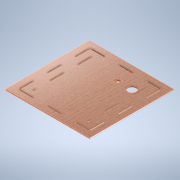
# Autodesk Inventor part: Roof_V2
Saved by Autodesk Inventor 2022.2 (Build 262287000, 287)
## iProperties
Created: 2022-11-15
Part Number: Roof_V2
Material: Generic
Document SubType Name: Modeling
Designer: jaege
Density: 1 g/cm^3
Appearance: Red Oak - Natural Low Gloss
Mass: 344.053 g
Surface Area: 1843.39 cm^2
Volume: 344.053 cm^3
Author: jaege
Autodesk Inventor part; units mm, degrees
(part 1 of 2)
ref_plane "YZ Plane" through (0, 0, 0) normal (1, 0, 0) x (0, 1, 0)
ref_plane "XZ Plane" through (0, 0, 0) normal (0, 1, 0) x (-1, 0, 0)
ref_plane "XY Plane" through (0, 0, 0) normal (0, 0, 1) x (1, 0, 0)
sketch "Sketch1" plane through (0, 0, 0) normal (0, 0, 1) x (1, 0, 0)
  line L0 (120, -66) -> (20, -66) construction
  line L1 (20, -66) -> (20, -26) construction
  line L2 (20, -26) -> (120, -26) construction
  line L3 (120, -26) -> (120, -66) construction
  line L4 (-275, -71) -> (125, -71) construction
  line L5 (125, -71) -> (125, 329) construction
  line L6 (125, 329) -> (-275, 329) construction
  line L7 (-275, 329) -> (-275, -71) construction
  line L8 (50, 104) -> (50, 154) construction
  line L9 (50, 154) -> (54, 154) construction
  line L10 (54, 154) -> (54, 104) construction
  line L11 (54, 104) -> (50, 104) construction
  line L12 (-50, 254) -> (-100, 254) construction
  line L13 (-100, 254) -> (-100, 258) construction
  line L14 (-100, 258) -> (-50, 258) construction
  line L15 (-50, 258) -> (-50, 254) construction
  line L16 (50, 258) -> (50, 254) construction
  line L17 (50, 254) -> (54, 254) construction
  line L18 (54, 254) -> (54, 204) construction
  line L19 (54, 204) -> (50, 204) construction
  line L20 (50, 204) -> (50, 254) construction
  line L21 (50, 254) -> (0, 254) construction
  line L22 (0, 254) -> (0, 258) construction
  line L23 (0, 258) -> (50, 258) construction
  line L24 (54, 4) -> (50, 4) construction
  line L25 (50, 4) -> (50, 0) construction
  line L26 (50, 0) -> (0, 0) construction
  line L27 (0, 0) -> (0, 4) construction
  line L28 (0, 4) -> (50, 4) construction
  line L29 (50, 4) -> (50, 54) construction
  line L30 (50, 54) -> (54, 54) construction
  line L31 (54, 54) -> (54, 4) construction
  line L32 (-100, 4) -> (-50, 4) construction
  line L33 (-50, 4) -> (-50, 0) construction
  line L34 (-50, 0) -> (-100, 0) construction
  line L35 (-100, 0) -> (-100, 4) construction
  line L36 (-204, 254) -> (-200, 254) construction
  line L37 (-200, 254) -> (-200, 258) construction
  line L38 (-200, 258) -> (-150, 258) construction
  line L39 (-150, 258) -> (-150, 254) construction
  line L40 (-150, 254) -> (-200, 254) construction
  line L41 (-200, 254) -> (-200, 204) construction
  line L42 (-200, 204) -> (-204, 204) construction
  line L43 (-204, 204) -> (-204, 254) construction
  line L44 (-200, 154) -> (-200, 104) construction
  line L45 (-200, 104) -> (-204, 104) construction
  line L46 (-204, 104) -> (-204, 154) construction
  line L47 (-204, 154) -> (-200, 154) construction
  line L48 (-200, 54) -> (-200, 4) construction
  line L49 (-200, 4) -> (-150, 4) construction
  line L50 (-150, 4) -> (-150, 0) construction
  line L51 (-150, 0) -> (-200, 0) construction
  line L52 (-200, 0) -> (-200, 4) construction
  line L53 (-200, 4) -> (-204, 4) construction
  line L54 (-204, 4) -> (-204, 54) construction
  line L55 (-204, 54) -> (-200, 54) construction
  line L56 (-275, -71) -> (125, -71) construction
  line L57 (125, -71) -> (125, 329) construction
  line L58 (125, 329) -> (-275, 329) construction
  line L59 (-275, 329) -> (-275, -71) construction
  line L60 (-275, -71) -> (125, 329) construction
  line L61 (75, 279) -> (-225, 279)
  line L62 (-225, 279) -> (-225, -21)
  line L63 (-225, -21) -> (75, -21)
  line L64 (75, -21) -> (75, 279)
  line L65 (75, 279) -> (-225, -21) construction
  line L66 (-225, 279) -> (75, -21) construction
  line L67 (-204, 4) -> (-200, 4)
  line L68 (-200, 4) -> (-200, 54)
  line L69 (-200, 54) -> (-204, 54)
  line L70 (-204, 54) -> (-204, 4)
  line L71 (-200, 104) -> (-204, 104)
  line L72 (-204, 104) -> (-204, 154)
  line L73 (-204, 154) -> (-200, 154)
  line L74 (-200, 154) -> (-200, 104)
  line L75 (-200, 204) -> (-204, 204)
  line L76 (-204, 204) -> (-204, 254)
  line L77 (-204, 254) -> (-200, 254)
  line L78 (-200, 254) -> (-200, 204)
  line L79 (-200, 254) -> (-150, 254)
  line L80 (-150, 254) -> (-150, 258)
  line L81 (-150, 258) -> (-200, 258)
  line L82 (-200, 258) -> (-200, 254)
  line L83 (-100, 254) -> (-50, 254)
  line L84 (-50, 254) -> (-50, 258)
  line L85 (-50, 258) -> (-100, 258)
  line L86 (-100, 258) -> (-100, 254)
  line L87 (0, 254) -> (50, 254)
  line L88 (50, 254) -> (50, 258)
  line L89 (50, 258) -> (0, 258)
  line L90 (0, 258) -> (0, 254)
  line L91 (50, 254) -> (54, 254)
  line L92 (54, 254) -> (54, 204)
  line L93 (54, 204) -> (50, 204)
  line L94 (50, 204) -> (50, 254)
  line L95 (54, 154) -> (50, 154)
  line L96 (50, 154) -> (50, 104)
  line L97 (50, 104) -> (54, 104)
  line L98 (54, 104) -> (54, 154)
  line L99 (54, 4) -> (50, 4)
  line L100 (50, 4) -> (50, 54)
  line L101 (50, 54) -> (54, 54)
  line L102 (54, 54) -> (54, 4)
  line L103 (50, 4) -> (0, 4)
  line L104 (0, 4) -> (0, 0)
  line L105 (0, 0) -> (50, 0)
  line L106 (50, 0) -> (50, 4)
  line L107 (-100, 0) -> (-50, 0)
  line L108 (-50, 0) -> (-50, 4)
  line L109 (-50, 4) -> (-100, 4)
  line L110 (-100, 4) -> (-100, 0)
  line L111 (-200, 0) -> (-150, 0)
  line L112 (-150, 0) -> (-150, 4)
  line L113 (-150, 4) -> (-200, 4)
  line L114 (-200, 4) -> (-200, 0)
  point P0 (-75, 129)
  dimension "d0" = 300
  dimension "d1" = 300
  constraints: 118 end point, 28 parallel, 14 horizontal, 14 perpendicular, 3 midpoint
  measures "d0" distance of L63.end L62.end
  measures "d1" distance of L62.end L61.end
extrude "Extrusion1" add sketch "Sketch1" against normal blind 4
sketch "Sketch2" plane through (0, 0, 0) normal (0, 0, 1) x (1, 0, 0)
  line L0 (-175, 234) -> (-171, 234)
  line L1 (-171, 234) -> (-171, 184)
  line L2 (-171, 184) -> (-175, 184)
  line L3 (-175, 184) -> (-175, 234)
  line L4 (-175, 184) -> (-171, 184)
  line L5 (-171, 184) -> (-171, 134)
  line L6 (-171, 134) -> (-175, 134)
  line L7 (-175, 134) -> (-175, 184)
  line L8 (-175, 134) -> (-171, 134)
  line L9 (-171, 134) -> (-171, 84)
  line L10 (-171, 84) -> (-175, 84)
  line L11 (-175, 84) -> (-175, 134)
  line L12 (-200, 254) -> (-200, 204) projected
  line L13 (-150, 254) -> (-200, 254) projected
  line L14 (-175, 84) -> (-171, 84)
  line L15 (-171, 84) -> (-171, 34)
  line L16 (-171, 34) -> (-175, 34)
  line L17 (-175, 34) -> (-175, 84)
  line L18 (-175, 34) -> (-171, 34)
  line L19 (-171, 34) -> (-171, 24)
  line L20 (-171, 24) -> (-175, 24)
  line L21 (-175, 24) -> (-175, 34)
  line L22 (-200, 4) -> (-150, 4) projected
  line L23 (25, 184) -> (21, 184)
  line L24 (21, 184) -> (25, 184)
  line L25 (21, 234) -> (25, 234)
  line L26 (25, 234) -> (25, 184)
  line L27 (21, 184) -> (21, 234)
  line L28 (25, 184) -> (25, 134)
  line L29 (25, 134) -> (21, 134)
  line L30 (21, 134) -> (25, 134)
  line L31 (25, 134) -> (25, 84)
  line L32 (25, 84) -> (21, 84)
  line L33 (21, 84) -> (21, 134)
  line L34 (21, 134) -> (21, 184)
  line L35 (21, 84) -> (25, 84)
  line L36 (25, 84) -> (25, 34)
  line L37 (21, 34) -> (21, 84)
  line L38 (25, 34) -> (21, 34)
  line L39 (21, 34) -> (25, 34)
  line L40 (25, 34) -> (25, 24)
  line L41 (21, 24) -> (21, 34)
  line L42 (25, 24) -> (21, 24)
  circle A0 centre (0, 204) radius 15
  line L43 (50, 254) -> (0, 254) projected
  line L44 (50, 204) -> (50, 254) projected
  point P0 (0, 0)
  point P1 (-173, 234)
  point P2 (-173, 24)
  point P3 (23, 234)
  point P4 (23, 24)
  point P5 (23, 234)
  point P6 (-75, 184)
  dimension "d4" = 4
  dimension "d5" = 50
  dimension "d6" = 4
  dimension "d7" = 50
  dimension "d8" = 4
  dimension "d9" = 50
  dimension "d10" = 25
  dimension "d11" = 20
  dimension "d12" = 4
  dimension "d13" = 50
  dimension "d14" = 4
  dimension "d15" = 20
  dimension "d20" = 196
  dimension "d25" = 30
  dimension "d29" = 50
  dimension "d30" = 50
  constraints: 80 end point, 10 parallel, 6 horizontal, 5 perpendicular, 3 midpoint, 1 centre point, 38 other
  measures "d4" distance of L1.end L2.end
  measures "d5" distance of L0.end L1.end
  measures "d6" distance of L5.end L6.end
  measures "d7" distance of L4.end L5.end
  measures "d8" distance of L9.end L10.end
  measures "d9" distance of L8.end L9.end
  measures "d10" distance from line of L12 L0.start
  measures "d11" distance from line of L13 point (-173, 234)
  measures "d12" distance of L15.end L16.end
  measures "d13" distance of L14.end L15.end
  measures "d14" distance of L19.end L20.end
  measures "d15" distance from line of L22 point (-173, 24)
  measures "d20" distance of L2.end L23.end
  measures "d25" diameter of A0
  measures "d29" distance of L43.end A0.centre
  measures "d30" distance from line of L44 A0.centre
extrude "Extrusion2" cut sketch "Sketch2" against normal blind 10 contours L0 L1 L2 L3 | L6 L9 L10 L11 | L16 L19 L20 L21 | L23 L27 L25 L26 | L31 L32 L33 L29 | L40 L42 L41 L38 | A0
sketch "Sketch3" plane through (0, 0, 0) normal (0, 0, 1) x (1, 0, 0)
  circle A0 centre (-50, 204) radius 6
  line L0 (-50, 254) -> (-100, 254) projected
  circle A1 centre (0, 204) radius 15 projected
  point P0 (0, 0)
  dimension "d31" = 12
  dimension "d32" = 50
  dimension "d33" = 50
  constraints: 1 centre point
  measures "d31" diameter of A0
  measures "d32" distance from line of A0.centre L0
  measures "d33" distance of A1.centre A0.centre
extrude "Extrusion3" cut sketch "Sketch3" against normal through all contours A0
sketch "Sketch4" plane through (0, 0, 0) normal (0, 0, 1) x (1, 0, 0)
  circle A0 centre (-50, 204) radius 6 projected
  line L0 (21, 84) -> (21, 134) projected
  line L1 (21, 134) -> (25, 134) projected
  line L2 (25, 134) -> (25, 84) projected
  line L3 (25, 84) -> (21, 84) projected
  line L4 (-175, 24) -> (-175, 34) projected
  line L5 (-175, 34) -> (-171, 34) projected
  line L6 (-171, 34) -> (-171, 24) projected
  line L7 (-171, 24) -> (-175, 24) projected
  line L8 (21, 24) -> (21, 34) projected
  line L9 (21, 34) -> (25, 34) projected
  line L10 (25, 34) -> (25, 24) projected
  line L11 (25, 24) -> (21, 24) projected
  line L12 (21, 184) -> (21, 234) projected
  line L13 (21, 234) -> (25, 234) projected
  line L14 (25, 234) -> (25, 184) projected
  line L15 (25, 184) -> (21, 184) projected
  line L16 (-175, 84) -> (-175, 134) projected
  line L17 (-175, 134) -> (-171, 134) projected
  line L18 (-171, 134) -> (-171, 84) projected
  line L19 (-171, 84) -> (-175, 84) projected
  line L20 (-175, 184) -> (-175, 234) projected
  line L21 (-175, 234) -> (-171, 234) projected
  line L22 (-171, 234) -> (-171, 184) projected
  line L23 (-171, 184) -> (-175, 184) projected
  circle A1 centre (0, 204) radius 15 projected
  line L24 (-225, 279) -> (-225, -21) projected
  line L25 (-225, -21) -> (75, -21) projected
  line L26 (75, -21) -> (75, 279) projected
  line L27 (75, 279) -> (-225, 279) projected
  line L28 (-100, 0) -> (-100, 4) projected
  line L29 (-100, 4) -> (-50, 4) projected
  line L30 (-50, 4) -> (-50, 0) projected
  line L31 (-50, 0) -> (-100, 0) projected
  line L32 (54, 4) -> (50, 4) projected
  line L33 (50, 4) -> (50, 0) projected
  line L34 (50, 0) -> (0, 0) projected
  line L35 (0, 0) -> (0, 4) projected
  line L36 (0, 4) -> (50, 4) projected
  line L37 (50, 4) -> (50, 54) projected
  line L38 (50, 54) -> (54, 54) projected
  line L39 (54, 54) -> (54, 4) projected
  line L40 (54, 154) -> (54, 104) projected
  line L41 (54, 104) -> (50, 104) projected
  line L42 (50, 104) -> (50, 154) projected
  line L43 (50, 154) -> (54, 154) projected
  line L44 (50, 204) -> (50, 254) projected
  line L45 (50, 254) -> (0, 254) projected
  line L46 (0, 254) -> (0, 258) projected
  line L47 (0, 258) -> (50, 258) projected
  line L48 (50, 258) -> (50, 254) projected
  line L49 (50, 254) -> (54, 254) projected
  line L50 (54, 254) -> (54, 204) projected
  line L51 (54, 204) -> (50, 204) projected
  line L52 (-100, 254) -> (-100, 258) projected
  line L53 (-100, 258) -> (-50, 258) projected
  line L54 (-50, 258) -> (-50, 254) projected
  line L55 (-50, 254) -> (-100, 254) projected
  line L56 (-204, 254) -> (-200, 254) projected
  line L57 (-200, 254) -> (-200, 258) projected
  line L58 (-200, 258) -> (-150, 258) projected
  line L59 (-150, 258) -> (-150, 254) projected
  line L60 (-150, 254) -> (-200, 254) projected
  line L61 (-200, 254) -> (-200, 204) projected
  line L62 (-200, 204) -> (-204, 204) projected
  line L63 (-204, 204) -> (-204, 254) projected
  line L64 (-200, 104) -> (-204, 104) projected
  line L65 (-204, 104) -> (-204, 154) projected
  line L66 (-204, 154) -> (-200, 154) projected
  line L67 (-200, 154) -> (-200, 104) projected
  line L68 (-200, 54) -> (-200, 4) projected
  line L69 (-200, 4) -> (-150, 4) projected
  line L70 (-150, 4) -> (-150, 0) projected
  line L71 (-150, 0) -> (-200, 0) projected
  line L72 (-200, 0) -> (-200, 4) projected
  line L73 (-200, 4) -> (-204, 4) projected
  line L74 (-204, 4) -> (-204, 54) projected
  line L75 (-204, 54) -> (-200, 54) projected
  line L76 (-58.1443, 209.9414) -> (-57.4426, 209.0769)
  line L77 (-57.4426, 209.0769) -> (-57.732, 208.6915)
  line L78 (-57.732, 208.6915) -> (-60.2646, 209.6927)
  spline S0 degree 2 poles (-60.2646, 209.6927) (-60.3488, 209.7261) (-60.425, 209.7304) (-60.4722, 209.7028) knots 0 0 0 1 2 2 2
  spline S1 degree 2 poles (-60.4722, 209.7028) (-60.5537, 209.6515) (-60.6194, 209.7008) knots 0 0 0 1 1 1
  spline S2 degree 2 poles (-60.6194, 209.7008) (-60.6723, 209.7406) (-60.6606, 209.8708) (-60.6002, 209.9513) knots 0 0 0 1 2 2 2
  line L79 (-60.6002, 209.9513) -> (-59.9722, 210.7875)
  spline S3 degree 2 poles (-59.9722, 210.7875) (-59.9134, 210.8659) (-59.8716, 210.8775) knots 0 0 0 1 1 1
  spline S4 degree 2 poles (-59.8716, 210.8775) (-59.8154, 210.895) (-59.7689, 210.86) knots 0 0 0 1 1 1
  spline S5 degree 2 poles (-59.7689, 210.86) (-59.7138, 210.8186) (-59.7218, 210.7286) knots 0 0 0 1 1 1
  spline S6 degree 2 poles (-59.7218, 210.7286) (-59.7319, 210.6534) (-59.7139, 210.5936) (-59.6716, 210.5618) knots 0 0 0 1 2 2 2
  spline S7 degree 2 poles (-59.6716, 210.5618) (-59.6525, 210.5475) (-59.6287, 210.5395) knots 0 0 0 1 1 1
  line L80 (-59.6287, 210.5395) -> (-58.1443, 209.9414)
  line L81 (-59.5923, 211.2936) -> (-59.3157, 211.6619)
  line L82 (-59.3157, 211.6619) -> (-57.367, 210.8708)
  line L83 (-57.367, 210.8708) -> (-56.7066, 210.0571)
  line L84 (-56.7066, 210.0571) -> (-56.9991, 209.6676)
  line L85 (-56.9991, 209.6676) -> (-58.8832, 210.4301)
  line L86 (-58.8832, 210.4301) -> (-59.5923, 211.2936)
  line L87 (-57.6019, 211.1532) -> (-58.0339, 211.3319)
  line L88 (-58.0339, 211.3319) -> (-58.4646, 211.8606)
  spline S8 degree 2 poles (-58.4646, 211.8606) (-58.5154, 211.9252) (-58.5493, 211.9506) knots 0 0 0 1 1 1
  spline S9 degree 2 poles (-58.5493, 211.9506) (-58.6022, 211.9904) (-58.723, 211.9883) (-58.8077, 211.946) knots 0 0 0 1 2 2 2
  spline S10 degree 2 poles (-58.8077, 211.946) (-58.866, 211.9169) (-58.9359, 211.9164) (-58.9697, 211.9419) knots 0 0 0 1 2 2 2
  spline S11 degree 2 poles (-58.9697, 211.9419) (-59.0163, 211.9768) (-59.012, 212.0663) (-58.9643, 212.1298) knots 0 0 0 1 2 2 2
  line L89 (-58.9643, 212.1298) -> (-58.6448, 212.5554)
  spline S12 degree 2 poles (-58.6448, 212.5554) (-58.5892, 212.6295) (-58.5044, 212.6586) (-58.4557, 212.622) knots 0 0 0 1 2 2 2
  spline S13 degree 2 poles (-58.4557, 212.622) (-58.4261, 212.5997) (-58.4124, 212.5431) (-58.4225, 212.4944) knots 0 0 0 1 2 2 2
  spline S14 degree 2 poles (-58.4225, 212.4944) (-58.4469, 212.3869) (-58.4353, 212.3186) knots 0 0 0 1 1 1
  spline S15 degree 2 poles (-58.4353, 212.3186) (-58.4168, 212.1756) (-58.2903, 212.0177) knots 0 0 0 1 1 1
  line L90 (-58.2903, 212.0177) -> (-57.6019, 211.1532)
  line L91 (-56.7345, 213.9981) -> (-55.9742, 214.48)
  line L92 (-55.9742, 214.48) -> (-54.045, 212.5932)
  spline S16 degree 2 poles (-54.045, 212.5932) (-53.9924, 212.545) (-53.9462, 212.5116) knots 0 0 0 1 1 1
  spline S17 degree 2 poles (-53.9462, 212.5116) (-53.9056, 212.4872) (-53.8333, 212.5017) knots 0 0 0 1 1 1
  spline S18 degree 2 poles (-53.8333, 212.5017) (-53.77, 212.5105) (-53.7064, 212.4943) (-53.6838, 212.4585) knots 0 0 0 1 2 2 2
  spline S19 degree 2 poles (-53.6838, 212.4585) (-53.6214, 212.3601) (-53.769, 212.2666) knots 0 0 0 1 1 1
  line L93 (-53.769, 212.2666) -> (-54.7105, 211.6699)
  spline S20 degree 2 poles (-54.7105, 211.6699) (-54.7664, 211.6345) (-54.8711, 211.6465) (-54.8995, 211.6912) knots 0 0 0 1 2 2 2
  spline S21 degree 2 poles (-54.8995, 211.6912) (-54.9236, 211.7292) (-54.9164, 211.7871) (-54.8819, 211.8465) knots 0 0 0 1 2 2 2
  spline S22 degree 2 poles (-54.8819, 211.8465) (-54.8567, 211.8907) (-54.8537, 211.9553) (-54.875, 211.9888) knots 0 0 0 1 2 2 2
  spline S23 degree 2 poles (-54.875, 211.9888) (-54.8962, 212.0224) (-54.9185, 212.0427) knots 0 0 0 1 1 1
  line L94 (-54.9185, 212.0427) -> (-55.1518, 212.2773)
  line L95 (-55.1518, 212.2773) -> (-55.6773, 211.9442)
  line L96 (-55.6773, 211.9442) -> (-55.7676, 212.2004)
  line L97 (-55.7676, 212.2004) -> (-55.345, 212.4683)
  line L98 (-55.345, 212.4683) -> (-56.6661, 213.7813)
  line L99 (-56.6661, 213.7813) -> (-56.7345, 213.9981)
  line L100 (-56.5617, 213.4337) -> (-56.219, 213.1055)
  line L101 (-56.219, 213.1055) -> (-55.7798, 211.6756)
  spline S24 degree 2 poles (-55.7798, 211.6756) (-55.7614, 211.612) (-55.7331, 211.5672) knots 0 0 0 1 1 1
  spline S25 degree 2 poles (-55.7331, 211.5672) (-55.6579, 211.4487) (-55.5135, 211.4681) knots 0 0 0 1 1 1
  line L102 (-55.5135, 211.4681) -> (-55.4288, 211.4779)
  spline S26 degree 2 poles (-55.4288, 211.4779) (-55.3492, 211.4908) (-55.3067, 211.4237) knots 0 0 0 1 1 1
  spline S27 degree 2 poles (-55.3067, 211.4237) (-55.2472, 211.3298) (-55.3836, 211.2433) knots 0 0 0 1 1 1
  line L103 (-55.3836, 211.2433) -> (-55.8621, 210.94)
  spline S28 degree 2 poles (-55.8621, 210.94) (-55.9337, 210.8947) (-56.0511, 210.9018) (-56.0837, 210.9532) knots 0 0 0 1 2 2 2
  spline S29 degree 2 poles (-56.0837, 210.9532) (-56.1177, 211.0069) (-56.0576, 211.0951) knots 0 0 0 1 1 1
  spline S30 degree 2 poles (-56.0576, 211.0951) (-56.002, 211.1805) (-55.9622, 211.2809) (-55.9585, 211.3492) knots 0 0 0 1 2 2 2
  spline S31 degree 2 poles (-55.9585, 211.3492) (-55.9566, 211.46) (-56.0016, 211.6102) knots 0 0 0 1 1 1
  line L104 (-56.0016, 211.6102) -> (-56.5617, 213.4337)
  line L105 (-52.9721, 215.6794) -> (-52.3659, 213.1239)
  spline S32 degree 2 poles (-52.3659, 213.1239) (-52.3457, 213.0389) (-52.3036, 213.0108) knots 0 0 0 1 1 1
  spline S33 degree 2 poles (-52.3036, 213.0108) (-52.2833, 212.9938) (-52.2493, 212.9883) (-52.1594, 212.9878) knots 0 0 0 1 2 2 2
  spline S34 degree 2 poles (-52.1594, 212.9878) (-52.0483, 212.9897) (-52.0257, 212.8944) knots 0 0 0 1 1 1
  spline S35 degree 2 poles (-52.0257, 212.8944) (-52.0123, 212.8377) (-52.0604, 212.7882) knots 0 0 0 1 1 1
  spline S36 degree 2 poles (-52.0604, 212.7882) (-52.0955, 212.7527) (-52.1908, 212.7301) knots 0 0 0 1 1 1
  line L106 (-52.1908, 212.7301) -> (-52.2655, 212.7123)
  line L107 (-52.2655, 212.7123) -> (-53.2367, 212.4819)
  line L108 (-53.2367, 212.4819) -> (-53.2934, 212.4685)
  spline S37 degree 2 poles (-53.2934, 212.4685) (-53.3706, 212.4502) (-53.4697, 212.4892) (-53.4825, 212.5433) knots 0 0 0 1 2 2 2
  spline S38 degree 2 poles (-53.4825, 212.5433) (-53.5033, 212.6309) (-53.4224, 212.68) knots 0 0 0 1 1 1
  spline S39 degree 2 poles (-53.4224, 212.68) (-53.3564, 212.7229) (-53.3357, 212.7387) (-53.3277, 212.7624) knots 0 0 0 1 2 2 2
  spline S40 degree 2 poles (-53.3277, 212.7624) (-53.3099, 212.802) (-53.3282, 212.8793) knots 0 0 0 1 1 1
  line L109 (-53.3282, 212.8793) -> (-53.844, 215.0535)
  spline S41 degree 2 poles (-53.844, 215.0535) (-53.8623, 215.1308) (-53.896, 215.1581) knots 0 0 0 1 1 1
  spline S42 degree 2 poles (-53.896, 215.1581) (-53.9138, 215.1757) (-53.9394, 215.1805) (-54.0171, 215.1866) knots 0 0 0 1 2 2 2
  spline S43 degree 2 poles (-54.0171, 215.1866) (-54.1114, 215.1941) (-54.1328, 215.2843) knots 0 0 0 1 1 1
  spline S44 degree 2 poles (-54.1328, 215.2843) (-54.1456, 215.3384) (-54.0747, 215.4178) (-53.9974, 215.4361) knots 0 0 0 1 2 2 2
  line L110 (-53.9974, 215.4361) -> (-53.9407, 215.4496)
  line L111 (-53.9407, 215.4496) -> (-52.9721, 215.6794)
  spline S45 degree 2 poles (-51.9455, 214.3229) (-51.7405, 214.3416) (-51.5064, 214.3183) (-51.4035, 214.2746) knots 0 0 0 1 2 2 2
  spline S46 degree 2 poles (-51.4035, 214.2746) (-51.2974, 214.2291) (-51.1555, 214.0668) (-51.1305, 213.9612) knots 0 0 0 1 2 2 2
  line L112 (-51.1305, 213.9612) -> (-51.0242, 213.5129)
  spline S47 degree 2 poles (-51.0242, 213.5129) (-51.007, 213.4408) (-50.9607, 213.4518) knots 0 0 0 1 1 1
  spline S48 degree 2 poles (-50.9607, 213.4518) (-50.9452, 213.4555) (-50.9243, 213.4822) (-50.9105, 213.5154) knots 0 0 0 1 2 2 2
  spline S49 degree 2 poles (-50.9105, 213.5154) (-50.8741, 213.603) (-50.8174, 213.6164) knots 0 0 0 1 1 1
  spline S50 degree 2 poles (-50.8174, 213.6164) (-50.7813, 213.625) (-50.6883, 213.5654) (-50.6785, 213.5242) knots 0 0 0 1 2 2 2
  spline S51 degree 2 poles (-50.6785, 213.5242) (-50.6626, 213.4572) (-50.7456, 213.2335) (-50.8226, 213.1336) knots 0 0 0 1 2 2 2
  spline S52 degree 2 poles (-50.8226, 213.1336) (-50.8937, 213.0432) (-51.0871, 212.9293) (-51.2287, 212.8957) knots 0 0 0 1 2 2 2
  spline S53 degree 2 poles (-51.2287, 212.8957) (-51.5147, 212.8279) (-51.9149, 213.0812) (-51.984, 213.3723) knots 0 0 0 1 2 2 2
  line L113 (-51.984, 213.3723) -> (-52.0708, 213.7381)
  spline S54 degree 2 poles (-52.0708, 213.7381) (-52.0995, 213.8592) (-52.1069, 213.8792) knots 0 0 0 1 1 1
  spline S55 degree 2 poles (-52.1069, 213.8792) (-52.138, 213.9643) (-52.2042, 214.0139) knots 0 0 0 1 1 1
  spline S56 degree 2 poles (-52.2042, 214.0139) (-52.2844, 214.0766) (-52.4059, 214.0613) knots 0 0 0 1 1 1
  line L114 (-52.4059, 214.0613) -> (-52.4609, 214.2932)
  spline S57 degree 2 poles (-52.4609, 214.2932) (-52.3467, 214.3393) (-52.3082, 214.3947) knots 0 0 0 1 1 1
  spline S58 degree 2 poles (-52.3082, 214.3947) (-52.2735, 214.4437) (-52.2639, 214.5522) (-52.2871, 214.65) knots 0 0 0 1 2 2 2
  line L115 (-52.2871, 214.65) -> (-52.424, 215.2271)
  spline S59 degree 2 poles (-52.424, 215.2271) (-52.4564, 215.3636) (-52.5938, 215.4725) (-52.7421, 215.4782) knots 0 0 0 1 2 2 2
  line L116 (-52.7421, 215.4782) -> (-52.7995, 215.7203)
  line L117 (-52.7995, 215.7203) -> (-52.7428, 215.7338)
  spline S60 degree 2 poles (-52.7428, 215.7338) (-52.5033, 215.7906) (-52.329, 215.8129) knots 0 0 0 1 1 1
  spline S61 degree 2 poles (-52.329, 215.8129) (-52.071, 215.8496) (-51.839, 215.755) knots 0 0 0 1 1 1
  spline S62 degree 2 poles (-51.839, 215.755) (-51.508, 215.6213) (-51.4188, 215.2452) knots 0 0 0 1 1 1
  spline S63 degree 2 poles (-51.4188, 215.2452) (-51.346, 214.9386) (-51.4902, 214.6976) knots 0 0 0 1 1 1
  spline S64 degree 2 poles (-51.4902, 214.6976) (-51.5505, 214.5962) (-51.7425, 214.4418) (-51.9455, 214.3229) knots 0 0 0 1 2 2 2
  line L118 (-48.7411, 215.9844) -> (-47.7904, 213.7994)
  line L119 (-47.7904, 213.7994) -> (-47.9004, 212.8207)
  line L120 (-47.9004, 212.8207) -> (-48.5055, 212.8887)
  line L121 (-48.5055, 212.8887) -> (-49.7213, 215.6549)
  spline S65 degree 2 poles (-49.7213, 215.6549) (-49.7615, 215.7474) (-49.8172, 215.8202) (-49.8628, 215.8414) knots 0 0 0 1 2 2 2
  line L122 (-49.8628, 215.8414) -> (-49.9435, 215.8824)
  spline S66 degree 2 poles (-49.9435, 215.8824) (-49.9765, 215.8968) (-50.0095, 215.9591) (-50.0056, 215.9933) knots 0 0 0 1 2 2 2
  spline S67 degree 2 poles (-50.0056, 215.9933) (-50.0012, 216.0327) (-49.9546, 216.0914) (-49.9189, 216.1008) knots 0 0 0 1 2 2 2
  spline S68 degree 2 poles (-49.9189, 216.1008) (-49.8803, 216.1124) (-49.7119, 216.0935) knots 0 0 0 1 1 1
  line L123 (-49.7119, 216.0935) -> (-48.7411, 215.9844)
  line L124 (-49.7603, 215.3076) -> (-49.5699, 214.8919)
  line L125 (-49.5699, 214.8919) -> (-49.7035, 213.7027)
  spline S69 degree 2 poles (-49.7035, 213.7027) (-49.721, 213.5475) (-49.6382, 213.3357) (-49.5325, 213.2572) knots 0 0 0 1 2 2 2
  line L126 (-49.5325, 213.2572) -> (-49.4708, 213.213)
  spline S70 degree 2 poles (-49.4708, 213.213) (-49.4168, 213.1723) (-49.4242, 213.1065) knots 0 0 0 1 1 1
  spline S71 degree 2 poles (-49.4242, 213.1065) (-49.4298, 213.0565) (-49.4757, 213.027) knots 0 0 0 1 1 1
  spline S72 degree 2 poles (-49.4757, 213.027) (-49.5158, 213.0022) (-49.6263, 213.0147) knots 0 0 0 1 1 1
  line L127 (-49.6263, 213.0147) -> (-50.1367, 213.072)
  spline S73 degree 2 poles (-50.1367, 213.072) (-50.3393, 213.0948) (-50.3263, 213.2106) knots 0 0 0 1 1 1
  spline S74 degree 2 poles (-50.3263, 213.2106) (-50.3219, 213.25) (-50.2745, 213.2926) (-50.199, 213.3241) knots 0 0 0 1 2 2 2
  spline S75 degree 2 poles (-50.199, 213.3241) (-49.9726, 213.4186) (-49.9377, 213.729) knots 0 0 0 1 1 1
  line L128 (-49.9377, 213.729) -> (-49.7603, 215.3076)
  line L129 (-47.7505, 214.1546) -> (-47.94, 214.5782)
  line L130 (-47.94, 214.5782) -> (-47.8708, 215.1939)
  spline S76 degree 2 poles (-47.8708, 215.1939) (-47.8498, 215.3807) (-47.9355, 215.5901) (-48.067, 215.6768) knots 0 0 0 1 2 2 2
  spline S77 degree 2 poles (-48.067, 215.6768) (-48.1093, 215.7029) (-48.1403, 215.7597) (-48.1358, 215.7991) knots 0 0 0 1 2 2 2
  spline S78 degree 2 poles (-48.1358, 215.7991) (-48.129, 215.8596) (-48.0439, 215.906) (-47.9571, 215.8963) knots 0 0 0 1 2 2 2
  line L131 (-47.9571, 215.8963) -> (-47.4045, 215.8342)
  spline S79 degree 2 poles (-47.4045, 215.8342) (-47.2914, 215.8215) (-47.2587, 215.7805) knots 0 0 0 1 1 1
  spline S80 degree 2 poles (-47.2587, 215.7805) (-47.2257, 215.7421) (-47.2313, 215.6922) knots 0 0 0 1 1 1
  spline S81 degree 2 poles (-47.2313, 215.6922) (-47.2364, 215.6474) (-47.2838, 215.6048) (-47.3672, 215.5742) knots 0 0 0 1 2 2 2
  spline S82 degree 2 poles (-47.3672, 215.5742) (-47.4923, 215.527) (-47.5668, 215.4101) knots 0 0 0 1 1 1
  spline S83 degree 2 poles (-47.5668, 215.4101) (-47.6192, 215.3228) (-47.6366, 215.1676) knots 0 0 0 1 1 1
  line L132 (-47.6366, 215.1676) -> (-47.7505, 214.1546)
  line L133 (-46.1874, 212.1678) -> (-47.1139, 212.5393)
  line L134 (-47.1139, 212.5393) -> (-47.168, 212.561)
  spline S84 degree 2 poles (-47.168, 212.561) (-47.2417, 212.5905) (-47.3001, 212.6796) (-47.2794, 212.7312) knots 0 0 0 1 2 2 2
  spline S85 degree 2 poles (-47.2794, 212.7312) (-47.2459, 212.8147) (-47.1515, 212.8082) knots 0 0 0 1 1 1
  spline S86 degree 2 poles (-47.1515, 212.8082) (-47.0729, 212.8052) (-47.0468, 212.8062) (-47.0266, 212.8209) knots 0 0 0 1 2 2 2
  spline S87 degree 2 poles (-47.0266, 212.8209) (-46.9893, 212.843) (-46.9597, 212.9167) knots 0 0 0 1 1 1
  line L135 (-46.9597, 212.9167) -> (-46.1281, 214.9908)
  spline S88 degree 2 poles (-46.1281, 214.9908) (-46.0986, 215.0645) (-46.1103, 215.1063) knots 0 0 0 1 1 1
  spline S89 degree 2 poles (-46.1103, 215.1063) (-46.1147, 215.1309) (-46.1329, 215.1496) (-46.1928, 215.1993) knots 0 0 0 1 2 2 2
  spline S90 degree 2 poles (-46.1928, 215.1993) (-46.2656, 215.2598) (-46.2311, 215.3458) knots 0 0 0 1 1 1
  spline S91 degree 2 poles (-46.2311, 215.3458) (-46.2104, 215.3974) (-46.1066, 215.4215) (-46.0329, 215.3919) knots 0 0 0 1 2 2 2
  line L136 (-46.0329, 215.3919) -> (-45.9788, 215.3702)
  line L137 (-45.9788, 215.3702) -> (-45.0524, 214.9988)
  line L138 (-45.0524, 214.9988) -> (-44.9983, 214.9771)
  spline S92 degree 2 poles (-44.9983, 214.9771) (-44.9246, 214.9475) (-44.8662, 214.8585) (-44.8869, 214.8069) knots 0 0 0 1 2 2 2
  spline S93 degree 2 poles (-44.8869, 214.8069) (-44.9214, 214.7209) (-45.0157, 214.7273) knots 0 0 0 1 1 1
  spline S94 degree 2 poles (-45.0157, 214.7273) (-45.0934, 214.7328) (-45.1195, 214.7319) (-45.1396, 214.7171) knots 0 0 0 1 2 2 2
  spline S95 degree 2 poles (-45.1396, 214.7171) (-45.177, 214.695) (-45.2066, 214.6213) knots 0 0 0 1 1 1
  line L139 (-45.2066, 214.6213) -> (-46.0382, 212.5473)
  spline S96 degree 2 poles (-46.0382, 212.5473) (-46.0677, 212.4735) (-46.056, 212.4317) knots 0 0 0 1 1 1
  spline S97 degree 2 poles (-46.056, 212.4317) (-46.0516, 212.4072) (-46.0334, 212.3885) (-45.9744, 212.3363) knots 0 0 0 1 2 2 2
  spline S98 degree 2 poles (-45.9744, 212.3363) (-45.9017, 212.2758) (-45.9352, 212.1922) knots 0 0 0 1 1 1
  spline S99 degree 2 poles (-45.9352, 212.1922) (-45.9559, 212.1406) (-46.0597, 212.1166) (-46.1334, 212.1462) knots 0 0 0 1 2 2 2
  line L140 (-46.1334, 212.1462) -> (-46.1874, 212.1678)
  line L141 (-42.77, 213.6404) -> (-43.0752, 211.2772)
  line L142 (-43.0752, 211.2772) -> (-43.6718, 210.4936)
  line L143 (-43.6718, 210.4936) -> (-44.1563, 210.8625)
  line L144 (-44.1563, 210.8625) -> (-43.7803, 213.8606)
  spline S100 degree 2 poles (-43.7803, 213.8606) (-43.7674, 213.9606) (-43.7779, 214.0517) (-43.8062, 214.0932) knots 0 0 0 1 2 2 2
  line L145 (-43.8062, 214.0932) -> (-43.8544, 214.1698)
  spline S101 degree 2 poles (-43.8544, 214.1698) (-43.8753, 214.1991) (-43.8716, 214.2695) (-43.8508, 214.2969) knots 0 0 0 1 2 2 2
  spline S102 degree 2 poles (-43.8508, 214.2969) (-43.8267, 214.3285) (-43.7566, 214.355) (-43.7212, 214.3447) knots 0 0 0 1 2 2 2
  spline S103 degree 2 poles (-43.7212, 214.3447) (-43.6821, 214.3348) (-43.5473, 214.2322) knots 0 0 0 1 1 1
  line L146 (-43.5473, 214.2322) -> (-42.77, 213.6404)
  line L147 (-43.992, 213.5825) -> (-44.0419, 213.128)
  line L148 (-44.0419, 213.128) -> (-44.7669, 212.1759)
  spline S104 degree 2 poles (-44.7669, 212.1759) (-44.8615, 212.0516) (-44.8991, 211.8273) (-44.8486, 211.7057) knots 0 0 0 1 2 2 2
  line L149 (-44.8486, 211.7057) -> (-44.8184, 211.6361)
  spline S105 degree 2 poles (-44.8184, 211.6361) (-44.7929, 211.5735) (-44.833, 211.5208) knots 0 0 0 1 1 1
  spline S106 degree 2 poles (-44.833, 211.5208) (-44.8635, 211.4808) (-44.918, 211.479) knots 0 0 0 1 1 1
  spline S107 degree 2 poles (-44.918, 211.479) (-44.9652, 211.4783) (-45.0536, 211.5457) knots 0 0 0 1 1 1
  line L150 (-45.0536, 211.5457) -> (-45.4623, 211.8568)
  spline S108 degree 2 poles (-45.4623, 211.8568) (-45.6245, 211.9803) (-45.5539, 212.073) knots 0 0 0 1 1 1
  spline S109 degree 2 poles (-45.5539, 212.073) (-45.5299, 212.1046) (-45.4673, 212.1169) (-45.3864, 212.1052) knots 0 0 0 1 2 2 2
  spline S110 degree 2 poles (-45.3864, 212.1052) (-45.1436, 212.07) (-44.9543, 212.3186) knots 0 0 0 1 1 1
  line L151 (-44.9543, 212.3186) -> (-43.992, 213.5825)
  line L152 (-42.8586, 211.5616) -> (-42.8039, 212.0224)
  line L153 (-42.8039, 212.0224) -> (-42.4286, 212.5153)
  spline S111 degree 2 poles (-42.4286, 212.5153) (-42.3148, 212.6649) (-42.2809, 212.8886) (-42.3492, 213.0305) knots 0 0 0 1 2 2 2
  spline S112 degree 2 poles (-42.3492, 213.0305) (-42.3722, 213.0746) (-42.3696, 213.1392) (-42.3455, 213.1708) knots 0 0 0 1 2 2 2
  spline S113 degree 2 poles (-42.3455, 213.1708) (-42.3087, 213.2193) (-42.2118, 213.2154) (-42.1423, 213.1625) knots 0 0 0 1 2 2 2
  line L154 (-42.1423, 213.1625) -> (-41.6999, 212.8257)
  spline S114 degree 2 poles (-41.6999, 212.8257) (-41.6093, 212.7567) (-41.6023, 212.7048) knots 0 0 0 1 1 1
  spline S115 degree 2 poles (-41.6023, 212.7048) (-41.5936, 212.6549) (-41.6241, 212.6149) knots 0 0 0 1 1 1
  spline S116 degree 2 poles (-41.6241, 212.6149) (-41.6514, 212.5791) (-41.7139, 212.5668) (-41.8012, 212.5833) knots 0 0 0 1 2 2 2
  spline S117 degree 2 poles (-41.8012, 212.5833) (-41.9329, 212.6071) (-42.0567, 212.5449) knots 0 0 0 1 1 1
  spline S118 degree 2 poles (-42.0567, 212.5449) (-42.1465, 212.4969) (-42.2412, 212.3726) knots 0 0 0 1 1 1
  line L155 (-42.2412, 212.3726) -> (-42.8586, 211.5616)
  line L156 (-40.0083, 210.8443) -> (-40.2144, 210.7048)
  spline S119 degree 2 poles (-40.2144, 210.7048) (-40.3637, 210.8404) (-40.583, 210.6921) knots 0 0 0 1 1 1
  line L157 (-40.583, 210.6921) -> (-42.3067, 209.5262)
  spline S120 degree 2 poles (-42.3067, 209.5262) (-42.4054, 209.4595) (-42.4409, 209.3939) knots 0 0 0 1 1 1
  spline S121 degree 2 poles (-42.4409, 209.3939) (-42.4685, 209.3401) (-42.4473, 209.2426) knots 0 0 0 1 1 1
  line L158 (-42.4473, 209.2426) -> (-42.6578, 209.1002)
  spline S122 degree 2 poles (-42.6578, 209.1002) (-42.6978, 209.1594) (-42.7449, 209.2714) (-42.7734, 209.3704) knots 0 0 0 1 2 2 2
  spline S123 degree 2 poles (-42.7734, 209.3704) (-42.836, 209.6094) (-42.7754, 210.1106) (-42.6529, 210.3405) knots 0 0 0 1 2 2 2
  spline S124 degree 2 poles (-42.6529, 210.3405) (-42.4636, 210.6986) (-42.0557, 210.9745) knots 0 0 0 1 1 1
  spline S125 degree 2 poles (-42.0557, 210.9745) (-41.6609, 211.2415) (-40.8614, 211.3732) (-40.508, 211.2287) knots 0 0 0 1 2 2 2
  spline S126 degree 2 poles (-40.508, 211.2287) (-40.3047, 211.1456) (-40.1437, 211.002) knots 0 0 0 1 1 1
  spline S127 degree 2 poles (-40.1437, 211.002) (-40.075, 210.943) (-40.0083, 210.8443) knots 0 0 0 1 1 1
  spline S128 degree 2 poles (-41.6084, 208.3237) (-41.7334, 208.3478) (-42.053, 208.4896) (-42.1711, 208.5696) knots 0 0 0 1 2 2 2
  spline S129 degree 2 poles (-42.1711, 208.5696) (-42.2773, 208.6416) (-42.4902, 208.8524) (-42.5525, 208.9445) knots 0 0 0 1 2 2 2
  line L159 (-42.5525, 208.9445) -> (-42.3419, 209.0869)
  spline S130 degree 2 poles (-42.3419, 209.0869) (-42.2939, 209.0395) (-42.221, 209.0121) (-42.1726, 209.0161) knots 0 0 0 1 2 2 2
  spline S131 degree 2 poles (-42.1726, 209.0161) (-42.0948, 209.0239) (-42.0071, 209.0832) knots 0 0 0 1 1 1
  line L160 (-42.0071, 209.0832) -> (-41.4654, 209.4496)
  spline S132 degree 2 poles (-41.4654, 209.4496) (-41.393, 209.4986) (-41.3816, 209.5478) knots 0 0 0 1 1 1
  spline S133 degree 2 poles (-41.3816, 209.5478) (-41.373, 209.5729) (-41.3783, 209.6044) (-41.4119, 209.6872) knots 0 0 0 1 2 2 2
  spline S134 degree 2 poles (-41.4119, 209.6872) (-41.4508, 209.7919) (-41.3696, 209.8468) knots 0 0 0 1 1 1
  spline S135 degree 2 poles (-41.3696, 209.8468) (-41.3214, 209.8794) (-41.2124, 209.8317) (-41.1575, 209.7505) knots 0 0 0 1 2 2 2
  line L161 (-41.1575, 209.7505) -> (-41.116, 209.6891)
  line L162 (-41.116, 209.6891) -> (-40.6576, 209.0115)
  spline S136 degree 2 poles (-40.6576, 209.0115) (-40.6013, 208.9281) (-40.6014, 208.829) (-40.6584, 208.7904) knots 0 0 0 1 2 2 2
  spline S137 degree 2 poles (-40.6584, 208.7904) (-40.6935, 208.7667) (-40.7588, 208.7641) (-40.8103, 208.7836) knots 0 0 0 1 2 2 2
  spline S138 degree 2 poles (-40.8103, 208.7836) (-40.8619, 208.803) (-40.9176, 208.7909) (-40.9768, 208.7509) knots 0 0 0 1 2 2 2
  line L163 (-40.9768, 208.7509) -> (-41.6084, 208.3237)
  line L164 (-40.1077, 210.5565) -> (-39.9081, 210.6915)
  spline S139 degree 2 poles (-39.9081, 210.6915) (-39.7334, 210.3717) (-39.6847, 210.1202) knots 0 0 0 1 1 1
  spline S140 degree 2 poles (-39.6847, 210.1202) (-39.6725, 210.0454) (-39.6517, 210.0147) knots 0 0 0 1 1 1
  spline S141 degree 2 poles (-39.6517, 210.0147) (-39.631, 209.984) (-39.5817, 209.9725) (-39.4833, 209.9688) knots 0 0 0 1 2 2 2
  spline S142 degree 2 poles (-39.4833, 209.9688) (-39.415, 209.9671) (-39.3808, 209.9166) knots 0 0 0 1 1 1
  spline S143 degree 2 poles (-39.3808, 209.9166) (-39.3452, 209.864) (-39.3741, 209.7837) (-39.4421, 209.7378) knots 0 0 0 1 2 2 2
  line L165 (-39.4421, 209.7378) -> (-40.1614, 209.2512)
  spline S144 degree 2 poles (-40.1614, 209.2512) (-40.3039, 209.1548) (-40.3736, 209.2579) knots 0 0 0 1 1 1
  spline S145 degree 2 poles (-40.3736, 209.2579) (-40.4092, 209.3105) (-40.3885, 209.3981) (-40.32, 209.4764) knots 0 0 0 1 2 2 2
  spline S146 degree 2 poles (-40.32, 209.4764) (-40.2348, 209.5724) (-40.0563, 209.904) (-40.0219, 210.0232) knots 0 0 0 1 2 2 2
  spline S147 degree 2 poles (-40.0219, 210.0232) (-39.9795, 210.1638) (-40.0215, 210.4102) (-40.1077, 210.5565) knots 0 0 0 1 2 2 2
  line L166 (-41.6141, 195.3458) -> (-43.7131, 197.5586)
  line L167 (-43.7131, 197.5586) -> (-42.9908, 198.2437)
  line L168 (-42.9908, 198.2437) -> (-42.9486, 198.2838)
  spline S148 degree 2 poles (-42.9486, 198.2838) (-42.891, 198.3385) (-42.7857, 198.3544) (-42.7474, 198.3141) knots 0 0 0 1 2 2 2
  spline S149 degree 2 poles (-42.7474, 198.3141) (-42.6855, 198.2488) (-42.7307, 198.1657) knots 0 0 0 1 1 1
  spline S150 degree 2 poles (-42.7307, 198.1657) (-42.7663, 198.0954) (-42.7763, 198.0714) (-42.7713, 198.0469) knots 0 0 0 1 2 2 2
  spline S151 degree 2 poles (-42.7713, 198.0469) (-42.7668, 198.0037) (-42.7122, 197.9461) knots 0 0 0 1 1 1
  line L169 (-42.7122, 197.9461) -> (-41.1744, 196.3248)
  spline S152 degree 2 poles (-41.1744, 196.3248) (-41.1197, 196.2672) (-41.0768, 196.2605) knots 0 0 0 1 1 1
  spline S153 degree 2 poles (-41.0768, 196.2605) (-41.0526, 196.2542) (-41.0281, 196.2629) (-40.9579, 196.2967) knots 0 0 0 1 2 2 2
  spline S154 degree 2 poles (-40.9579, 196.2967) (-40.8725, 196.3375) (-40.8088, 196.2702) knots 0 0 0 1 1 1
  spline S155 degree 2 poles (-40.8088, 196.2702) (-40.7705, 196.2299) (-40.792, 196.1256) (-40.8496, 196.0709) knots 0 0 0 1 2 2 2
  line L170 (-40.8496, 196.0709) -> (-40.8919, 196.0308)
  line L171 (-40.8919, 196.0308) -> (-41.6141, 195.3458)
  spline S156 degree 2 poles (-43.1304, 195.9364) (-43.3038, 195.8267) (-43.5123, 195.7311) (-43.6138, 195.7151) knots 0 0 0 1 2 2 2
  spline S157 degree 2 poles (-43.6138, 195.7151) (-43.7907, 195.6823) (-44.1228, 195.8015) (-44.2558, 195.9418) knots 0 0 0 1 2 2 2
  spline S158 degree 2 poles (-44.2558, 195.9418) (-44.5182, 196.2184) (-44.4622, 196.5671) knots 0 0 0 1 1 1
  spline S159 degree 2 poles (-44.4622, 196.5671) (-44.433, 196.748) (-44.2413, 197.0576) (-44.0358, 197.2525) knots 0 0 0 1 2 2 2
  line L172 (-44.0358, 197.2525) -> (-43.8418, 197.4365)
  line L173 (-43.8418, 197.4365) -> (-43.6796, 197.2656)
  spline S160 degree 2 poles (-43.6796, 197.2656) (-43.7413, 197.1998) (-43.7907, 197.1018) (-43.7885, 197.0419) knots 0 0 0 1 2 2 2
  spline S161 degree 2 poles (-43.7885, 197.0419) (-43.784, 196.9294) (-43.6656, 196.8045) knots 0 0 0 1 1 1
  line L174 (-43.6656, 196.8045) -> (-43.3158, 196.4357)
  spline S162 degree 2 poles (-43.3158, 196.4357) (-43.2392, 196.355) (-43.1267, 196.2903) (-43.0538, 196.2865) knots 0 0 0 1 2 2 2
  spline S163 degree 2 poles (-43.0538, 196.2865) (-42.9976, 196.285) (-42.9106, 196.3201) (-42.8419, 196.367) knots 0 0 0 1 2 2 2
  line L175 (-42.8419, 196.367) -> (-42.6834, 196.1999)
  spline S164 degree 2 poles (-42.6834, 196.1999) (-42.7375, 196.1376) (-42.7809, 196.0526) (-42.7841, 196.0022) knots 0 0 0 1 2 2 2
  spline S165 degree 2 poles (-42.7841, 196.0022) (-42.7873, 195.9517) (-42.749, 195.8421) (-42.72, 195.8076) knots 0 0 0 1 2 2 2
  line L176 (-42.72, 195.8076) -> (-42.6343, 195.7173)
  line L177 (-42.6343, 195.7173) -> (-42.3683, 195.4368)
  spline S166 degree 2 poles (-42.3683, 195.4368) (-42.3264, 195.3927) (-42.2065, 195.324) (-42.1598, 195.3171) knots 0 0 0 1 2 2 2
  spline S167 degree 2 poles (-42.1598, 195.3171) (-42.0945, 195.3098) (-41.983, 195.3461) (-41.9123, 195.4023) knots 0 0 0 1 2 2 2
  line L178 (-41.9123, 195.4023) -> (-41.7428, 195.2237)
  line L179 (-41.7428, 195.2237) -> (-41.9311, 195.0451)
  spline S168 degree 2 poles (-41.9311, 195.0451) (-42.2999, 194.6953) (-42.6397, 194.6612) knots 0 0 0 1 1 1
  spline S169 degree 2 poles (-42.6397, 194.6612) (-42.7955, 194.6485) (-43.0773, 194.757) (-43.1866, 194.8723) knots 0 0 0 1 2 2 2
  spline S170 degree 2 poles (-43.1866, 194.8723) (-43.2941, 194.9856) (-43.3876, 195.2765) (-43.3649, 195.4257) knots 0 0 0 1 2 2 2
  spline S171 degree 2 poles (-43.3649, 195.4257) (-43.3507, 195.5377) (-43.2475, 195.7597) (-43.1304, 195.9364) knots 0 0 0 1 2 2 2
  line L180 (-44.8929, 195.4469) -> (-44.1793, 193.8489)
  spline S172 degree 2 poles (-44.1793, 193.8489) (-44.1469, 193.7764) (-44.1087, 193.7558) knots 0 0 0 1 1 1
  spline S173 degree 2 poles (-44.1087, 193.7558) (-44.088, 193.7418) (-44.0619, 193.7419) (-43.9845, 193.7504) knots 0 0 0 1 2 2 2
  spline S174 degree 2 poles (-43.9845, 193.7504) (-43.8904, 193.7605) (-43.8537, 193.6783) knots 0 0 0 1 1 1
  spline S175 degree 2 poles (-43.8537, 193.6783) (-43.83, 193.6251) (-43.8849, 193.5339) (-43.9574, 193.5015) knots 0 0 0 1 2 2 2
  line L181 (-43.9574, 193.5015) -> (-44.0106, 193.4777)
  line L182 (-44.0106, 193.4777) -> (-44.922, 193.0707)
  line L183 (-44.922, 193.0707) -> (-44.9752, 193.047)
  line L184 (-44.9752, 193.047) -> (-45.051, 193.0218)
  spline S176 degree 2 poles (-45.051, 193.0218) (-45.0902, 193.0188) (-45.1599, 193.0515) (-45.1761, 193.0878) knots 0 0 0 1 2 2 2
  spline S177 degree 2 poles (-45.1761, 193.0878) (-45.2128, 193.1699) (-45.1425, 193.2332) knots 0 0 0 1 1 1
  spline S178 degree 2 poles (-45.1425, 193.2332) (-45.0845, 193.2852) (-45.0671, 193.3046) (-45.0636, 193.3294) knots 0 0 0 1 2 2 2
  spline S179 degree 2 poles (-45.0636, 193.3294) (-45.0535, 193.3716) (-45.0859, 193.4441) knots 0 0 0 1 1 1
  line L185 (-45.0859, 193.4441) -> (-45.8502, 195.1557)
  spline S180 degree 2 poles (-45.8502, 195.1557) (-45.9269, 195.3273) (-46.0077, 195.4565) (-46.0592, 195.5002) knots 0 0 0 1 2 2 2
  spline S181 degree 2 poles (-46.0592, 195.5002) (-46.1084, 195.5391) (-46.1931, 195.5534) (-46.2979, 195.5414) knots 0 0 0 1 2 2 2
  line L186 (-46.2979, 195.5414) -> (-46.4178, 195.8098)
  line L187 (-46.4178, 195.8098) -> (-46.3743, 195.8292)
  spline S182 degree 2 poles (-46.3743, 195.8292) (-46.1083, 195.9479) (-45.9103, 195.9784) knots 0 0 0 1 1 1
  spline S183 degree 2 poles (-45.9103, 195.9784) (-45.681, 196.017) (-45.2744, 195.9376) (-45.1498, 195.8338) knots 0 0 0 1 2 2 2
  spline S184 degree 2 poles (-45.1498, 195.8338) (-45.0149, 195.7201) (-44.8929, 195.4469) knots 0 0 0 1 1 1
  line L188 (-46.6063, 195.7256) -> (-46.4865, 195.4572)
  spline S185 degree 2 poles (-46.4865, 195.4572) (-46.6777, 195.3399) (-46.7529, 195.1382) knots 0 0 0 1 1 1
  spline S186 degree 2 poles (-46.7529, 195.1382) (-46.8353, 194.9071) (-46.7014, 194.6074) knots 0 0 0 1 1 1
  line L189 (-46.7014, 194.6074) -> (-46.1076, 193.2778)
  spline S187 degree 2 poles (-46.1076, 193.2778) (-45.9824, 192.9973) (-45.7176, 192.9822) knots 0 0 0 1 1 1
  spline S188 degree 2 poles (-45.7176, 192.9822) (-45.6407, 192.9789) (-45.5804, 192.9478) (-45.561, 192.9043) knots 0 0 0 1 2 2 2
  spline S189 degree 2 poles (-45.561, 192.9043) (-45.5372, 192.8511) (-45.5941, 192.7706) (-45.6835, 192.7307) knots 0 0 0 1 2 2 2
  line L190 (-45.6835, 192.7307) -> (-46.1815, 192.5083)
  spline S190 degree 2 poles (-46.1815, 192.5083) (-46.2444, 192.4802) (-46.2911, 192.468) (-46.3159, 192.4715) knots 0 0 0 1 2 2 2
  spline S191 degree 2 poles (-46.3159, 192.4715) (-46.382, 192.4767) (-46.4057, 192.5299) knots 0 0 0 1 1 1
  spline S192 degree 2 poles (-46.4057, 192.5299) (-46.4263, 192.5758) (-46.4089, 192.6213) knots 0 0 0 1 1 1
  spline S193 degree 2 poles (-46.4089, 192.6213) (-46.4011, 192.6364) (-46.3432, 192.7144) knots 0 0 0 1 1 1
  spline S194 degree 2 poles (-46.3432, 192.7144) (-46.2764, 192.8051) (-46.2645, 193.0511) (-46.3228, 193.1817) knots 0 0 0 1 2 2 2
  line L191 (-46.3228, 193.1817) -> (-46.9165, 194.5113)
  spline S195 degree 2 poles (-46.9165, 194.5113) (-47.0698, 194.8546) (-47.0182, 195.1415) knots 0 0 0 1 1 1
  spline S196 degree 2 poles (-47.0182, 195.1415) (-46.9804, 195.3555) (-46.8181, 195.544) knots 0 0 0 1 1 1
  spline S197 degree 2 poles (-46.8181, 195.544) (-46.7392, 195.6401) (-46.6063, 195.7256) knots 0 0 0 1 1 1
  line L192 (-49.6882, 191.9034) -> (-49.7182, 192.1585)
  line L193 (-49.7182, 192.1585) -> (-48.8196, 195.0768)
  line L194 (-48.8196, 195.0768) -> (-47.8494, 195.1911)
  line L195 (-47.8494, 195.1911) -> (-47.8234, 194.9702)
  line L196 (-47.8234, 194.9702) -> (-48.7232, 192.0171)
  line L197 (-48.7232, 192.0171) -> (-49.6882, 191.9034)
  line L198 (-50.0449, 194.9325) -> (-49.0063, 195.0548)
  line L199 (-49.0063, 195.0548) -> (-49.0802, 194.8222)
  spline S198 degree 2 poles (-49.0802, 194.8222) (-49.3459, 194.7242) (-49.457, 194.6259) knots 0 0 0 1 1 1
  spline S199 degree 2 poles (-49.457, 194.6259) (-49.5535, 194.5398) (-49.66, 194.3353) (-49.7084, 194.135) knots 0 0 0 1 2 2 2
  spline S200 degree 2 poles (-49.7084, 194.135) (-49.7263, 194.061) (-49.7704, 194.0051) (-49.8151, 193.9998) knots 0 0 0 1 2 2 2
  spline S201 degree 2 poles (-49.8151, 193.9998) (-49.873, 193.993) (-49.9427, 194.0648) (-49.9517, 194.141) knots 0 0 0 1 2 2 2
  line L200 (-49.9517, 194.141) -> (-50.0449, 194.9325)
  line L201 (-47.5662, 192.1534) -> (-48.5286, 192.04)
  line L202 (-48.5286, 192.04) -> (-48.4479, 192.3054)
  spline S202 degree 2 poles (-48.4479, 192.3054) (-48.2617, 192.354) (-48.1172, 192.4857) knots 0 0 0 1 1 1
  spline S203 degree 2 poles (-48.1172, 192.4857) (-47.9338, 192.6486) (-47.8938, 192.9199) knots 0 0 0 1 1 1
  spline S204 degree 2 poles (-47.8938, 192.9199) (-47.8834, 192.9904) (-47.837, 193.0492) (-47.7871, 193.0551) knots 0 0 0 1 2 2 2
  spline S205 degree 2 poles (-47.7871, 193.0551) (-47.674, 193.0684) (-47.6588, 192.9396) knots 0 0 0 1 1 1
  line L203 (-47.6588, 192.9396) -> (-47.5662, 192.1534)
  line L204 (-52.8634, 192.2431) -> (-52.8257, 192.4971)
  line L205 (-52.8257, 192.4971) -> (-51.195, 195.0788)
  line L206 (-51.195, 195.0788) -> (-50.2286, 194.9353)
  line L207 (-50.2286, 194.9353) -> (-50.2613, 194.7153)
  line L208 (-50.2613, 194.7153) -> (-51.9023, 192.1003)
  line L209 (-51.9023, 192.1003) -> (-52.8634, 192.2431)
  line L210 (-52.4154, 195.26) -> (-51.3809, 195.1064)
  line L211 (-51.3809, 195.1064) -> (-51.5131, 194.9012)
  spline S206 degree 2 poles (-51.5131, 194.9012) (-51.7952, 194.8761) (-51.9281, 194.8102) knots 0 0 0 1 1 1
  spline S207 degree 2 poles (-51.9281, 194.8102) (-52.0437, 194.7525) (-52.2001, 194.583) (-52.2992, 194.4023) knots 0 0 0 1 2 2 2
  spline S208 degree 2 poles (-52.2992, 194.4023) (-52.3359, 194.3355) (-52.393, 194.2931) (-52.4375, 194.2997) knots 0 0 0 1 2 2 2
  spline S209 degree 2 poles (-52.4375, 194.2997) (-52.4951, 194.3083) (-52.5437, 194.3958) (-52.5324, 194.4717) knots 0 0 0 1 2 2 2
  line L212 (-52.5324, 194.4717) -> (-52.4154, 195.26)
  line L213 (-50.75, 191.9292) -> (-51.7085, 192.0716)
  line L214 (-51.7085, 192.0716) -> (-51.5611, 192.3066)
  spline S210 degree 2 poles (-51.5611, 192.3066) (-51.3687, 192.3048) (-51.1948, 192.3941) knots 0 0 0 1 1 1
  spline S211 degree 2 poles (-51.1948, 192.3941) (-50.9752, 192.5034) (-50.8656, 192.7547) knots 0 0 0 1 1 1
  spline S212 degree 2 poles (-50.8656, 192.7547) (-50.8372, 192.8201) (-50.777, 192.8647) (-50.7272, 192.8573) knots 0 0 0 1 2 2 2
  spline S213 degree 2 poles (-50.7272, 192.8573) (-50.6146, 192.8406) (-50.6337, 192.7123) knots 0 0 0 1 1 1
  line L215 (-50.6337, 192.7123) -> (-50.75, 191.9292)
  line L216 (-55.0547, 193.0613) -> (-53.7893, 195.8364)
  line L217 (-53.7893, 195.8364) -> (-52.8836, 195.4234)
  line L218 (-52.8836, 195.4234) -> (-52.8306, 195.3992)
  spline S214 degree 2 poles (-52.8306, 195.3992) (-52.7583, 195.3663) (-52.7041, 195.2746) (-52.7271, 195.224) knots 0 0 0 1 2 2 2
  spline S215 degree 2 poles (-52.7271, 195.224) (-52.7645, 195.1421) (-52.8585, 195.153) knots 0 0 0 1 1 1
  spline S216 degree 2 poles (-52.8585, 195.153) (-52.9369, 195.1596) (-52.963, 195.1599) (-52.9838, 195.1461) knots 0 0 0 1 2 2 2
  spline S217 degree 2 poles (-52.9838, 195.1461) (-53.0222, 195.1258) (-53.0551, 195.0535) knots 0 0 0 1 1 1
  line L219 (-53.0551, 195.0535) -> (-53.9822, 193.0203)
  spline S218 degree 2 poles (-53.9822, 193.0203) (-54.0152, 192.9481) (-54.0054, 192.9058) knots 0 0 0 1 1 1
  spline S219 degree 2 poles (-54.0054, 192.9058) (-54.0021, 192.881) (-53.9848, 192.8615) (-53.9273, 192.809) knots 0 0 0 1 2 2 2
  spline S220 degree 2 poles (-53.9273, 192.809) (-53.8574, 192.7452) (-53.8959, 192.6609) knots 0 0 0 1 1 1
  spline S221 degree 2 poles (-53.8959, 192.6609) (-53.9189, 192.6103) (-54.0237, 192.5911) (-54.096, 192.6241) knots 0 0 0 1 2 2 2
  line L220 (-54.096, 192.6241) -> (-54.149, 192.6483)
  line L221 (-54.149, 192.6483) -> (-55.0547, 193.0613)
  line L222 (-53.9724, 195.9199) -> (-54.0724, 195.7007)
  spline S222 degree 2 poles (-54.0724, 195.7007) (-54.2137, 195.7418) (-54.4212, 195.7462) (-54.5419, 195.7111) knots 0 0 0 1 2 2 2
  spline S223 degree 2 poles (-54.5419, 195.7111) (-54.6627, 195.6759) (-54.8399, 195.5618) (-54.9485, 195.4512) knots 0 0 0 1 2 2 2
  spline S224 degree 2 poles (-54.9485, 195.4512) (-54.9998, 195.3961) (-55.0689, 195.3723) (-55.1122, 195.3921) knots 0 0 0 1 2 2 2
  spline S225 degree 2 poles (-55.1122, 195.3921) (-55.1676, 195.4173) (-55.1827, 195.5056) (-55.1453, 195.5875) knots 0 0 0 1 2 2 2
  line L223 (-55.1453, 195.5875) -> (-54.818, 196.3054)
  line L224 (-54.818, 196.3054) -> (-53.9724, 195.9199)
  line L225 (-55.2354, 193.1437) -> (-56.0545, 193.5171)
  line L226 (-56.0545, 193.5171) -> (-55.726, 194.2374)
  spline S226 degree 2 poles (-55.726, 194.2374) (-55.6975, 194.3) (-55.624, 194.3335) (-55.571, 194.3093) knots 0 0 0 1 2 2 2
  spline S227 degree 2 poles (-55.571, 194.3093) (-55.5253, 194.2884) (-55.5008, 194.2336) (-55.5103, 194.1681) knots 0 0 0 1 2 2 2
  spline S228 degree 2 poles (-55.5103, 194.1681) (-55.5397, 193.8993) (-55.3542, 193.515) (-55.1267, 193.3821) knots 0 0 0 1 2 2 2
  line L227 (-55.1267, 193.3821) -> (-55.2354, 193.1437)
  line L228 (-54.5502, 194.6208) -> (-54.6579, 194.3847)
  spline S229 degree 2 poles (-54.6579, 194.3847) (-54.8023, 194.3807) (-54.977, 194.2974) (-55.054, 194.1987) knots 0 0 0 1 2 2 2
  spline S230 degree 2 poles (-55.054, 194.1987) (-55.1061, 194.1293) (-55.1865, 194.0932) (-55.2347, 194.1152) knots 0 0 0 1 2 2 2
  spline S231 degree 2 poles (-55.2347, 194.1152) (-55.2997, 194.1449) (-55.3008, 194.2064) knots 0 0 0 1 1 1
  spline S232 degree 2 poles (-55.3008, 194.2064) (-55.3031, 194.2395) (-55.2603, 194.3335) knots 0 0 0 1 1 1
  line L229 (-55.2603, 194.3335) -> (-54.9066, 195.1092)
  spline S233 degree 2 poles (-54.9066, 195.1092) (-54.8627, 195.2055) (-54.7863, 195.258) (-54.7309, 195.2327) knots 0 0 0 1 2 2 2
  spline S234 degree 2 poles (-54.7309, 195.2327) (-54.6828, 195.2108) (-54.6561, 195.1288) (-54.6724, 195.0548) knots 0 0 0 1 2 2 2
  spline S235 degree 2 poles (-54.6724, 195.0548) (-54.7, 194.8986) (-54.6404, 194.691) (-54.5502, 194.6208) knots 0 0 0 1 2 2 2
  line L230 (-58.0857, 195.0635) -> (-56.2922, 196.9821)
  spline S236 degree 2 poles (-56.2922, 196.9821) (-56.2325, 197.0459) (-56.2324, 197.0965) knots 0 0 0 1 1 1
  spline S237 degree 2 poles (-56.2324, 197.0965) (-56.2295, 197.1228) (-56.2437, 197.1542) (-56.293, 197.2293) knots 0 0 0 1 2 2 2
  spline S238 degree 2 poles (-56.293, 197.2293) (-56.3561, 197.3208) (-56.2892, 197.3924) knots 0 0 0 1 1 1